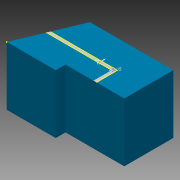
# Autodesk Inventor part: River1
Saved by Autodesk Inventor 2015 (Build 190159000, 159)
## iProperties
Created: 2015-08-24
Part Number: River1
Material: 一般
Document SubType Name: Modeling
Designer: nobuhiro
Density: 1 g/cm^3
Appearance: スカイ ブルー 標準
Author: nobuhiro
Autodesk Inventor part; units mm, degrees
ref_plane "YZ Plane" through (0, 0, 0) normal (1, 0, 0) x (0, 1, 0)
ref_plane "XZ Plane" through (0, 0, 0) normal (0, 1, 0) x (-1, 0, 0)
ref_plane "XY Plane" through (0, 0, 0) normal (0, 0, 1) x (1, 0, 0)
sketch "スケッチ1" plane through (0, 0, 0) normal (0, 0, 1) x (1, 0, 0)
  line L0 (0, 0) -> (-248.5281, 600)
  line L1 (-248.5281, 600) -> (-1100, 600)
  line L2 (-1100, 600) -> (-1100, 100)
  line L3 (-1100, 100) -> (-500, 100)
  line L4 (-500, 100) -> (-500, 0)
  line L5 (-500, 0) -> (0, 0)
  line L6 (0, 0) -> (0, 1201.6741) construction
  line L7 (0, 0) -> (248.5281, 600)
  line L8 (248.5281, 600) -> (1100, 600)
  line L9 (1100, 600) -> (1100, 100)
  line L10 (1100, 100) -> (500, 100)
  line L11 (500, 100) -> (500, 0)
  line L12 (500, 0) -> (0, 0)
  dimension "d0" = 67.5
  dimension "d2" = 600
  dimension "d3" = 100
  dimension "d4" = 1100
  dimension "d5" = 600
  constraints: 26 end point, 5 symmetric about line, 4 perpendicular, 1 horizontal, 1 vertical
  measures "d0" angle of L5 L0
  measures "d2" distance of L2.end L3.end
  measures "d3" distance of L3.end L4.end
  measures "d4" distance from line of L0.start L2
  measures "d5" distance between parallel lines of L5 L1
extrude "押し出し1" add sketch "スケッチ1" along normal blind 600 contours L7 L8 L9 L10 L11 L12
sketch "スケッチ2" plane through (0, 0, 600) normal (0, 0, 1) x (1, 0, 0)
  line L0 (118.0509, 285) -> (785, 285)
  line L1 (785, 285) -> (785, 315)
  line L2 (785, 315) -> (130.4773, 315)
  line L3 (130.4773, 315) -> (118.0509, 285)
  line L4 (815, 100) -> (785, 100)
  line L5 (785, 100) -> (785, 315)
  line L6 (785, 315) -> (815, 315)
  line L7 (815, 315) -> (815, 100)
  line L8 (500, 100) -> (1100, 100) projected
  line L9 (248.5281, 600) -> (0, 0) projected
  point P0 (800, 100)
  point P1 (800, 100)
  point P2 (124.2641, 300)
  point P3 (-147.2757, 300)
  point P4 (800, 100)
  point P5 (124.2641, 300)
  dimension "d8" = 30
  constraints: 16 end point, 4 midpoint, 3 coincident, 3 parallel, 3 perpendicular, 2 horizontal, 2 point on line, 1 horizontal alignment
  measures "d8" distance between parallel lines of L5 L7
extrude "押し出し2" add sketch "スケッチ2" along normal blind 0.1
sketch "スケッチ3" plane through (0, 0, 600.1) normal (0, 0, 1) x (1, 0, 0)
  line L0 (118.0509, 285) -> (785, 285) projected
  line L1 (815, 100) -> (815, 315) projected
  line L2 (815, 315) -> (130.4773, 315) projected
  point P0 (0, 0)
  point P1 (800, 300)
  point P2 (600, 300)
  dimension "d11" = 15
  dimension "d12" = 15
  dimension "d13" = 15
  dimension "d14" = 200
  measures "d11" distance from line of L0 point (800, 300)
  measures "d12" distance from line of point (800, 300) L1
  measures "d13" distance from line of point (600, 300) L2
  measures "d14" distance of point (800, 300) point (600, 300)
equation "\"d12\" = d11"
